tire v1 (Autodesk Fusion 360 design; units mm, degrees)
Autodesk Fusion 360 part; units mm, degrees
sketch "スケッチ1" plane through (0, 0, 0) normal (0, 1, 0) x (1, 0, 0)
  line L0 (0, 0) -> (5.4, 0)
  line L1 (5.4, 0) -> (5.4, -3.5)
  line L2 (5.4, -3.5) -> (6.55, -3.5)
  line L3 (6.55, -3.5) -> (6.8, -2.25)
  line L4 (6.8, -2.25) -> (6.8, -1.25)
  line L5 (6.8, -1.25) -> (6.55, 0)
  line L6 (6.55, 0) -> (5.4, 0)
  dimension "d1" = 3.5
  dimension "d3" = 5.4
  dimension "d4" = 1
  dimension "d5" = 0.25
  dimension "d8" = 6.8
  measures "d1" distance of L0.end L1.end
  measures "d3" distance of L0.start L0.end
  measures "d4" distance of L3.end L4.end
  measures "d5" distance of L4.end L5.end
  measures "d8" distance of L0.start L4
revolve "回転1" add sketch "スケッチ1" angle 360 about axis through (0, 0, 1.75) along (0, 0, 1)
fillet "フィレット1" radius 1 4 edges at (-6.1067, -2.3686, 0) (-6.3398, -2.459, 1.25) (-6.3398, -2.459, 2.25) (-6.1067, -2.3686, 3.5)
equation "d8 = ( 13.6 / 2 ) * 1 mm"
